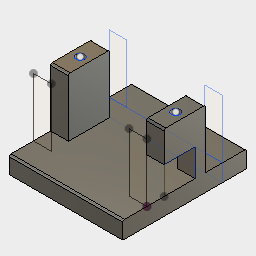
ServoBase v3 (Autodesk Fusion 360 design; units mm, degrees)
Autodesk Fusion 360 part; units mm, degrees
sketch "Sketch1" plane through (0, 0, 0) normal (0, 0, 1) x (1, 0, 0)
  line L0 (-13, 8) -> (20, 8)
  line L1 (20, 8) -> (20, 3)
  line L2 (20, 3) -> (-13, 3)
  line L3 (-13, 3) -> (-13, 8)
  line L4 (-13, 8) -> (-7.8, 8)
  line L5 (-7.8, 8) -> (-7.8, 25)
  line L6 (-7.8, 25) -> (-13, 25)
  line L7 (-13, 25) -> (-13, 8)
  line L8 (20, 8) -> (14.8, 8)
  line L9 (14.8, 8) -> (14.8, 25)
  line L10 (14.8, 25) -> (20, 25)
  line L11 (20, 25) -> (20, 8)
  dimension "d1" = 33
  dimension "d2" = 5
  dimension "d3" = 5.2
  dimension "d4" = 17
  dimension "d5" = 17
  dimension "d6" = 5.2
  measures "d1" distance of L0.start L0.end
  measures "d2" distance of L0.start L2.end
  measures "d3" distance of L0.start L4.end
  measures "d4" distance of L0.start L6.end
  measures "d5" distance of L0.end L10.end
  measures "d6" distance of L0.end L8.end
extrude "Extrude1" add sketch "Sketch1" along normal blind 22
sketch "Sketch2" plane through (0, 0, 22) normal (0, 0, 1) x (1, 0, 0)
  line L0 (-7.8, 8) -> (-7.8, 25)
  line L1 (-7.8, 25) -> (-13, 25)
  line L2 (-13, 25) -> (-13, 3)
  line L3 (-13, 3) -> (20, 3)
  line L4 (20, 3) -> (20, 25)
  line L5 (20, 25) -> (14.8, 25)
  line L6 (14.8, 25) -> (14.8, 8)
  line L7 (14.8, 8) -> (-7.8, 8)
  line L8 (-13, 25) -> (-7.8, 25)
  line L9 (-7.8, 25) -> (-7.8, 8)
  line L10 (-7.8, 8) -> (-13, 8)
  line L11 (-13, 8) -> (-13, 25)
  line L12 (14.8, 25) -> (20, 25)
  line L13 (20, 25) -> (20, 8)
  line L14 (20, 8) -> (14.8, 8)
  line L15 (14.8, 8) -> (14.8, 25)
  line L16 (20, 25) -> (14.8, 25)
  line L17 (14.8, 25) -> (14.8, 8)
  line L18 (14.8, 8) -> (20, 8)
  line L19 (20, 8) -> (20, 25)
  line L20 (-7.8, 25) -> (-13, 25)
  line L21 (-13, 25) -> (-13, 8)
  line L22 (-13, 8) -> (-7.8, 8)
  line L23 (-7.8, 8) -> (-7.8, 25)
  point P0 (20, 8)
  dimension "d9" = 17
  dimension "d10" = 5.2
  dimension "d15" = 5.2
  dimension "d16" = 17
  measures "d9" distance of L1.end L10.end
  measures "d10" distance of L1.end L0.end
  measures "d15" distance of L4.end L5.end
  measures "d16" distance of L4.end P0
extrude "Extrude5" cut sketch "Sketch1" along normal blind 5 contours L0 L4 L5 L6 L7
extrude "Extrude4" cut sketch "Sketch1" along normal blind 5 contours L0 L8 L9 L10 L11
extrude "Extrude3" cut sketch "Sketch2" against normal blind 5 contours L4 L5 L6 L12 L13 L14 L15 L16 L17 L18 L19
extrude "Extrude2" cut sketch "Sketch2" against normal blind 5 contours L0 L1 L2 L8 L9 L10 L11 L20 L21 L22 L23
extrude "Extrude6" add sketch "Sketch1" against normal blind 7 contours L0 L1 L2 L3 L4 L8
extrude "Extrude7" add sketch "Sketch2" along normal blind 7 contours L2 L3 L4 L7 L10 L14 L18 L22
sketch "Sketch3" plane through (20, 0, 0) normal (1, 0, 0) x (0, 0, -1)
  line L0 (-17, 25) -> (-17, 8)
  line L1 (-17, 8) -> (-29, 8)
  line L2 (-29, 8) -> (-29, 3)
  line L3 (-29, 3) -> (7, 3)
  line L4 (7, 3) -> (7, 8)
  line L5 (7, 8) -> (-5, 8)
  line L6 (-5, 8) -> (-5, 25)
  line L7 (-5, 25) -> (-17, 25)
  line L8 (-17, 8) -> (-8, 8)
  line L9 (-8, 8) -> (-8, 16)
  line L10 (-8, 16) -> (-17, 16)
  line L11 (-17, 16) -> (-17, 8)
extrude "Extrude8" cut sketch "Sketch3" against normal blind 9 contours L0 L8 L9 L10 L11
chamfer "Chamfer1" distance 0.5 angle 45 1 edges at (17.4, 25, 17)
fillet "Fillet1" radius 0.5 1 edges at (-10.4, 25, 17)
fillet "Fillet2" radius 0.5 1 edges at (-10.4, 25, 5)
fillet "Fillet3" radius 0.5 1 edges at (17.4, 25, 5)
fillet "Fillet4" radius 0.5 2 edges at (3.5, 8, 29) (3.5, 8, -7)
sketch "Sketch4" plane through (0, 25, 0) normal (0, 1, 0) x (-1, 0, 0)
  line L0 (7.8, 5.5) -> (13, 5.5)
  line L1 (13, 5.5) -> (13, 16.5)
  line L2 (13, 16.5) -> (7.8, 16.5)
  line L3 (7.8, 16.5) -> (7.8, 5.5)
  circle A0 centre (10.4, 11) radius 1.25
  circle A1 centre (-17.4, 11) radius 1.25
  dimension "d32" = 2.5
  dimension "d33" = 2.5
  measures "d32" diameter of A0
  measures "d33" diameter of A1
extrude "Extrude9" cut sketch "Sketch4" against normal blind 5 contours A0
extrude "Extrude10" cut sketch "Sketch4" against normal blind 5 contours A1
